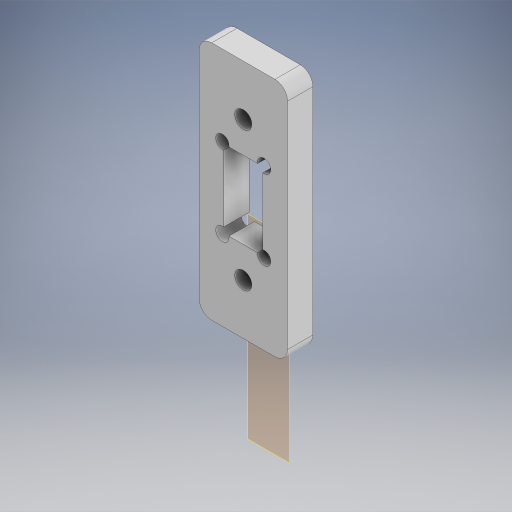
# Autodesk Inventor part: under the head_zig5
Saved by Autodesk Inventor 2024 (Build 280153000, 153)
## iProperties
Created: 2024-09-11
Part Number: under the head_zig5
Material: 일반
Document SubType Name: Modeling
Designer: ASUS
Density: 1 g/cm^3
Appearance: 기본값
Author: ASUS
Autodesk Inventor part; units mm, degrees
ref_plane "YZ Plane" through (0, 0, 0) normal (1, 0, 0) x (0, 1, 0)
ref_plane "XZ Plane" through (0, 0, 0) normal (0, 1, 0) x (-1, 0, 0)
ref_plane "XY Plane" through (0, 0, 0) normal (0, 0, 1) x (1, 0, 0)
ref_plane "작업 평면1" through (0, -41, 0) normal (0, 0, 1) x (1, 0, 0)
sketch "스케치1" plane through (0, -41, 0) normal (0, 0, 1) x (1, 0, 0)
  line L0 (0, 12) -> (0, 0) projected
  line L1 (0, 0) -> (6, 0) projected
  line L2 (6, 12) -> (6, 0) projected
  line L3 (0, 12) -> (6, 12) projected
  line L4 (6.3, -0.3) -> (-0.3, -0.3)
  line L5 (-0.3, -0.3) -> (-0.3, 12.3)
  line L6 (-0.3, 12.3) -> (6.3, 12.3)
  line L7 (6.3, 12.3) -> (6.3, -0.3)
  line L8 (0, 51) -> (6, 51) projected
  circle A0 centre (3, 17) radius 1.35 projected
  line L9 (0, -29) -> (6, -29) projected
  circle A1 centre (3, -5) radius 1.35 projected
  line L10 (10, 25) -> (-4, 25)
  line L11 (-4, 25) -> (-4, -13)
  line L12 (-4, -13) -> (10, -13)
  line L13 (10, -13) -> (10, 25)
  circle A2 centre (6.3, 12.3) radius 1.05
  circle A3 centre (-0.3, 12.3) radius 1.05
  circle A4 centre (-0.3, -0.3) radius 1.05
  circle A5 centre (6.3, -0.3) radius 1.05
  point P0 (0, 41)
  point P1 (0, -9)
  point P2 (5.25, -0.3)
  point P3 (0.75, -0.3)
  point P4 (-0.3, 0.75)
  point P5 (-0.3, 11.25)
  point P6 (0.75, 12.3)
  point P7 (5.25, 12.3)
  point P8 (6.3, 11.25)
  point P9 (6.3, 0.75)
  dimension "d0" = 0.3
  dimension "d2" = 2.1
  dimension "d3" = 2.1
  dimension "d4" = 2.1
  dimension "d5" = 2.1
  constraints: 16 end point, 4 centre point, 2 parallel, 1 coincident, 1 perpendicular, 3 other
  measures "d0" distance between parallel lines of L2 L7
  measures "d2" diameter of A2
  measures "d3" diameter of A3
  measures "d4" diameter of A4
  measures "d5" diameter of A5
extrude "돌출1" add sketch "스케치1" along normal blind 4
fillet "모깎기1" radius 2 4 edges at (10, -16, 2) (-4, -16, 2) (10, -54, 2) (-4, -54, 2)
sketch "스케치2" plane through (0, -41, 0) normal (0, 0, -1) x (-1, 0, 0)
  arc A0 (2, -13) -> (4, -11) centre (2, -11) ccw projected
  line L0 (4, 23) -> (4, -11) projected
  arc A1 (4, 23) -> (2, 25) centre (2, 23) ccw projected
  line L1 (-8, 25) -> (2, 25) projected
  arc A2 (-8, 25) -> (-10, 23) centre (-8, 23) ccw projected
  line L2 (-10, -11) -> (-10, 23) projected
  arc A3 (-10, -11) -> (-8, -13) centre (-8, -11) ccw projected
  line L3 (2, -13) -> (-8, -13) projected
  circle A4 centre (-3, -5) radius 1.35 projected
  circle A5 centre (-3, 17) radius 1.35 projected
  arc A6 (-6.3, 0.75) -> (-5.25, -0.3) centre (-6.3, -0.3) ccw projected
  line L4 (-6.3, 11.25) -> (-6.3, 0.75) projected
  arc A7 (-5.25, 12.3) -> (-6.3, 11.25) centre (-6.3, 12.3) ccw projected
  line L5 (-0.75, 12.3) -> (-5.25, 12.3) projected
  arc A8 (0.3, 11.25) -> (-0.75, 12.3) centre (0.3, 12.3) ccw projected
  line L6 (0.3, 0.75) -> (0.3, 11.25) projected
  arc A9 (-0.75, -0.3) -> (0.3, 0.75) centre (0.3, -0.3) ccw projected
  line L7 (-5.25, -0.3) -> (-0.75, -0.3) projected
  arc A10 (-0.5261, -0.1) -> (0.1, 0.5261) centre (0.3, -0.3) ccw
  line L8 (0.1, 0.5261) -> (0.1, 11.4739)
  arc A11 (0.1, 11.4739) -> (-0.5261, 12.1) centre (0.3, 12.3) ccw
  line L9 (-0.5261, 12.1) -> (-5.4739, 12.1)
  arc A12 (-5.4739, 12.1) -> (-6.1, 11.4739) centre (-6.3, 12.3) ccw
  line L10 (-6.1, 11.4739) -> (-6.1, 0.5261)
  arc A13 (-6.1, 0.5261) -> (-5.4739, -0.1) centre (-6.3, -0.3) ccw
  line L11 (-5.4739, -0.1) -> (-0.5261, -0.1)
  point P0 (0, 41)
  dimension "d9" = 0.2
  constraints: 8 end point, 8 point on circle, 4 centre point, 7 other
  measures "d9" distance between parallel lines of L7 L11
extrude "돌출2" add sketch "스케치2" against normal up to surface (4 mm away) contours L4 A7 L5 A8 L6 A9 L7 A6
sketch "스케치3" plane through (0, -41, 0) normal (0, 0, -1) x (-1, 0, 0)
  line L0 (-0.5261, -0.1) -> (-5.4739, -0.1) projected
  arc A0 (-6.1, 0.5261) -> (-5.4739, -0.1) centre (-6.3, -0.3) ccw projected
  line L1 (-6.1, 0.5261) -> (-6.1, 11.4739) projected
  arc A1 (-5.4739, 12.1) -> (-6.1, 11.4739) centre (-6.3, 12.3) ccw projected
  line L2 (-5.4739, 12.1) -> (-0.5261, 12.1) projected
  arc A2 (0.1, 11.4739) -> (-0.5261, 12.1) centre (0.3, 12.3) ccw projected
  line L3 (0.1, 11.4739) -> (0.1, 0.5261) projected
  arc A3 (-0.5261, -0.1) -> (0.1, 0.5261) centre (0.3, -0.3) ccw projected
  arc A4 (2, -13) -> (4, -11) centre (2, -11) ccw projected
  line L4 (4, 23) -> (4, -11) projected
  arc A5 (4, 23) -> (2, 25) centre (2, 23) ccw projected
  line L5 (-8, 25) -> (2, 25) projected
  arc A6 (-8, 25) -> (-10, 23) centre (-8, 23) ccw projected
  line L6 (-10, -11) -> (-10, 23) projected
  arc A7 (-10, -11) -> (-8, -13) centre (-8, -11) ccw projected
  line L7 (2, -13) -> (-8, -13) projected
  circle A8 centre (-3, -5) radius 1.35 projected
  circle A9 centre (-3, 17) radius 1.35 projected
  point P0 (0, 41)
hole "구멍1" at (6.3, -41.3, 0) at (-0.3, -41.3, 0) at (-0.3, -28.7, 0) at (6.3, -28.7, 0) direction (0, 0, 1) diameter 2.1 end through all
